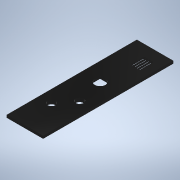
# Autodesk Inventor part: Arcade_ControlTop
Saved by Autodesk Inventor 2022 (Build 260153000, 153)
## iProperties
Created: 2023-12-22
Part Number: Arcade_ControlTop
Material: Generic
Document SubType Name: Modeling
Designer: Petr Černý
Density: 1 g/cm^3
Appearance: Smooth - Black
Author: Petr Černý
Autodesk Inventor part; units mm, degrees
ref_plane "YZ Plane" through (0, 0, 0) normal (1, 0, 0) x (0, 1, 0)
ref_plane "XZ Plane" through (0, 0, 0) normal (0, 1, 0) x (-1, 0, 0)
ref_plane "XY Plane" through (0, 0, 0) normal (0, 0, 1) x (1, 0, 0)
sketch "Sketch1" plane through (0, 0, 0) normal (0, 1, 0) x (-1, 0, 0)
  line L0 (23.5265, 54.5795) -> (-113.4735, 54.5795)
  line L1 (-113.4735, 54.5795) -> (-113.4735, -435.4205)
  line L2 (-113.4735, -435.4205) -> (23.5265, -435.4205)
  line L3 (23.5265, -435.4205) -> (23.5265, 54.5795)
  point P0 (0, 0)
  dimension "d0" = 137
  dimension "d1" = 490
  constraints: 8 end point, 2 parallel, 1 horizontal, 1 perpendicular
  measures "d0" distance of L2.end L1.end
  measures "d1" distance of L1.end L0.end
extrude "Extrusion1" add sketch "Sketch1" along normal blind 15
sketch "Sketch2" plane through (-23.5265, 0, 54.5795) normal (0, 0, 1) x (1, 0, 0)
  line L0 (137, 0) -> (0, 0) projected
  line L1 (0, 0) -> (127, 0)
  line L2 (127, 0) -> (127, 5)
  line L3 (127, 5) -> (0, 5)
  line L4 (0, 5) -> (0, 0)
  point P0 (23.5265, 0)
  dimension "d4" = 127
  dimension "d5" = 5
  constraints: 8 end point, 2 parallel, 1 horizontal, 1 perpendicular
  measures "d4" distance of L3.end L2.end
  measures "d5" distance of L2.end L1.end
extrude "Extrusion2" cut sketch "Sketch2" against normal blind 7
sketch "Sketch3" plane through (113.4735, 0, -435.4205) normal (0, 0, -1) x (-1, 0, 0)
  line L0 (0, 0) -> (137, 0) projected
  line L1 (0, 0) -> (137, 0)
  line L2 (137, 0) -> (137, 5)
  line L3 (137, 5) -> (0, 5)
  line L4 (0, 5) -> (0, 0)
  point P0 (113.4735, 0)
  dimension "d8" = 137
  dimension "d9" = 5
  constraints: 8 end point, 2 parallel, 1 horizontal, 1 perpendicular
  measures "d8" distance of L3.end L2.end
  measures "d9" distance of L2.end L1.end
extrude "Extrusion3" cut sketch "Sketch3" against normal blind 7
sketch "Sketch4" plane through (0, 0, 0) normal (0, -1, 0) x (1, 0, 0)
  line L0 (-23.5265, -428.4205) -> (113.4735, -428.4205) projected
  line L1 (103.4735, 47.5795) -> (-23.5265, 47.5795) projected
  line L2 (113.4735, -428.4205) -> (103.4735, -428.4205)
  line L3 (103.4735, -428.4205) -> (103.4735, 47.5795)
  line L4 (103.4735, 47.5795) -> (113.4735, 47.5795)
  line L5 (113.4735, 47.5795) -> (113.4735, -428.4205)
  point P0 (0, 0)
  point P1 (-13.5265, -428.4205)
  dimension "d12" = 10
  dimension "d13" = 476
  constraints: 8 end point, 2 parallel, 1 horizontal, 1 perpendicular
  measures "d12" distance of L1.start L4.end
  measures "d13" distance of L2.end L1.start
extrude "Extrusion4" cut sketch "Sketch4" against normal blind 5
sketch "Sketch5" plane through (0, 15, 0) normal (0, 1, 0) x (1, 0, 0)
  circle A0 centre (22.1402, 68.4205) radius 15
  circle A1 centre (67.8068, 128.4205) radius 15
  circle A2 centre (44.9735, 228.4205) radius 20
  line L0 (103.4735, 428.4205) -> (-23.5265, 428.4205) projected
  line L1 (-23.5265, 435.4205) -> (-23.5265, -54.5795) projected
  point P0 (0, 0)
  point P1 (-13.5265, 428.4205)
  dimension "d16" = 40
  dimension "d17" = 200
  dimension "d18" = 68.5
  dimension "d19" = 300
  dimension "d20" = 91.3333
  dimension "d21" = 45.6667
  dimension "d22" = 360
  dimension "d23" = 30
  dimension "d24" = 30
  constraints: 3 centre point
  measures "d16" diameter of A2
  measures "d17" distance from line of L0 A2.centre
  measures "d18" distance from line of A2.centre L1
  measures "d19" distance from line of L0 A1.centre
  measures "d20" distance from line of A1.centre L1
  measures "d21" distance from line of L1 A0.centre
  measures "d22" distance from line of L0 A0.centre
  measures "d23" diameter of A0
  measures "d24" diameter of A1
extrude "Extrusion5" cut sketch "Sketch5" against normal blind 15
sketch "Sketch6" plane through (0, 0, 0) normal (0, -1, 0) x (1, 0, 0)
  line L0 (69.9735, -253.4205) -> (19.9735, -253.4205)
  line L1 (19.9735, -253.4205) -> (19.9735, -203.4205)
  line L2 (19.9735, -203.4205) -> (69.9735, -203.4205)
  line L3 (69.9735, -203.4205) -> (69.9735, -253.4205)
  circle A0 centre (44.9735, -228.4205) radius 20 projected
  point P0 (0, 0)
  dimension "d27" = 25
  dimension "d28" = 50
  dimension "d29" = 25
  dimension "d30" = 50
  constraints: 8 end point, 2 parallel, 1 horizontal, 1 perpendicular
  measures "d27" distance from line of A0.centre L3
  measures "d28" distance of L0.start L0.end
  measures "d29" distance from line of L0 A0.centre
  measures "d30" distance between parallel lines of L2 L0
extrude "Extrusion6" cut sketch "Sketch6" against normal blind 12
sketch "Sketch7" plane through (0, 15, 0) normal (0, 1, 0) x (1, 0, 0)
  circle A0 centre (44.9735, 228.4205) radius 20 projected
  point P0 (0, 0)
  point P1 (28.7235, 212.1705)
  point P2 (28.7235, 244.6705)
  point P3 (61.2235, 244.6705)
  point P4 (61.2235, 212.1705)
  dimension "d33" = 16.25
  dimension "d34" = 16.25
  dimension "d35" = 16.25
  dimension "d36" = 16.25
  dimension "d37" = 16.25
  dimension "d38" = 16.25
  dimension "d39" = 16.25
  dimension "d40" = 16.25
  measures "d33" horizontal distance of A0.centre point (28.723, 212.17)
  measures "d34" horizontal distance of point (28.723, 244.67) A0.centre
  measures "d35" horizontal distance of A0.centre point (28.723, 244.67)
  measures "d36" horizontal distance of point (61.223, 244.67) A0.centre
  measures "d37" horizontal distance of A0.centre point (61.223, 244.67)
  measures "d38" horizontal distance of point (61.223, 212.17) A0.centre
  measures "d39" horizontal distance of A0.centre point (61.223, 212.17)
  measures "d40" horizontal distance of point (28.723, 212.17) A0.centre
hole "Hole1" at (28.7235, 15, -212.1705) at (28.7235, 15, -244.6705) at (61.2235, 15, -244.6705) at (61.2235, 15, -212.1705) direction (0, -1, 0) diameter 2.5 end through all
sketch "Sketch8" plane through (0, 0, 0) normal (0, -1, 0) x (1, 0, 0)
  circle A0 centre (61.2235, -244.6705) radius 1.25 projected
  circle A1 centre (28.7235, -212.1705) radius 1.25 projected
  circle A2 centre (28.7235, -244.6705) radius 1.25 projected
  circle A3 centre (61.2235, -212.1705) radius 1.25 projected
  line L0 (19.9735, -203.4205) -> (69.9735, -203.4205) projected
  line L1 (19.9735, -253.4205) -> (19.9735, -203.4205) projected
  line L2 (69.9735, -253.4205) -> (19.9735, -253.4205) projected
  line L3 (69.9735, -203.4205) -> (69.9735, -253.4205) projected
  circle A4 centre (44.9735, -228.4205) radius 20 projected
  line L4 (69.9735, -203.4205) -> (69.9735, -253.4205) projected
  line L5 (69.9735, -253.4205) -> (79.9735, -253.4205)
  line L6 (79.9735, -253.4205) -> (79.9735, -203.4205)
  line L7 (79.9735, -203.4205) -> (69.9735, -203.4205)
  line L8 (69.9735, -203.4205) -> (69.9735, -253.4205)
  line L9 (79.9735, -203.4205) -> (19.9735, -203.4205)
  line L10 (19.9735, -203.4205) -> (19.9735, -193.4205)
  line L11 (19.9735, -193.4205) -> (79.9735, -193.4205)
  line L12 (79.9735, -193.4205) -> (79.9735, -203.4205)
  point P0 (0, 0)
  dimension "d48" = 10
  dimension "d49" = 50
  dimension "d50" = 60
  dimension "d51" = 10
  constraints: 16 end point, 4 parallel, 2 horizontal, 2 perpendicular
  measures "d48" distance of L7.end L6.end
  measures "d49" distance of L6.end L5.end
  measures "d50" distance of L10.end L11.end
  measures "d51" distance of L9.end L10.end
extrude "Extrusion7" cut sketch "Sketch8" against normal blind 12 contours L10 L11 L12 L7 L0 | L7 L6 L5 L3
sketch "Sketch9" plane through (0, 15, 0) normal (0, 1, 0) x (1, 0, 0)
  line L0 (43.4735, 338.4205) -> (83.4735, 338.4205)
  line L1 (83.4735, 338.4205) -> (83.4735, 398.4205)
  line L2 (83.4735, 398.4205) -> (43.4735, 398.4205)
  line L3 (43.4735, 398.4205) -> (43.4735, 338.4205)
  line L4 (103.4735, 428.4205) -> (-23.5265, 428.4205) projected
  line L5 (113.4735, -54.5795) -> (113.4735, 435.4205) projected
  line L6 (46.6735, 342.9072) -> (52.6735, 342.9072)
  line L7 (52.6735, 342.9072) -> (52.6735, 392.9072)
  line L8 (52.6735, 392.9072) -> (46.6735, 392.9072)
  line L9 (46.6735, 392.9072) -> (46.6735, 342.9072)
  line L10 (55.8735, 342.9072) -> (61.8735, 342.9072)
  line L11 (61.8735, 342.9072) -> (61.8735, 392.9072)
  line L12 (61.8735, 392.9072) -> (55.8735, 392.9072)
  line L13 (55.8735, 392.9072) -> (55.8735, 342.9072)
  line L14 (65.0735, 342.9072) -> (71.0735, 342.9072)
  line L15 (71.0735, 342.9072) -> (71.0735, 392.9072)
  line L16 (71.0735, 392.9072) -> (65.0735, 392.9072)
  line L17 (65.0735, 392.9072) -> (65.0735, 342.9072)
  line L18 (74.2735, 342.9072) -> (80.2735, 342.9072)
  line L19 (80.2735, 342.9072) -> (80.2735, 392.9072)
  line L20 (80.2735, 392.9072) -> (74.2735, 392.9072)
  line L21 (74.2735, 392.9072) -> (74.2735, 342.9072)
  point P0 (0, 0)
  point P1 (-13.5265, 428.4205)
  dimension "d54" = 60
  dimension "d55" = 40
  dimension "d56" = 30
  dimension "d57" = 30
  dimension "d58" = 50
  dimension "d59" = 50
  dimension "d60" = 6
  dimension "d61" = 6
  dimension "d62" = 6
  dimension "d63" = 6
  dimension "d64" = 3.2
  dimension "d65" = 3.2
  dimension "d66" = 3.2
  dimension "d67" = 3.2
  constraints: 40 end point, 10 parallel, 5 horizontal, 5 perpendicular, 5 point on line
  measures "d54" distance of L2.end L0.start
  measures "d55" distance of L1.end L2.end
  measures "d56" distance between parallel lines of L4 L2
  measures "d57" distance between parallel lines of L5 L1
  measures "d58" distance of L8.end L6.start
  measures "d59" distance of L12.end L10.start
  measures "d60" distance of L7.end L8.end
  measures "d61" distance of L11.end L12.end
  measures "d62" distance of L15.end L16.end
  measures "d63" distance between parallel lines of L19 L21
  measures "d64" distance between parallel lines of L9 L3
  measures "d65" distance between parallel lines of L13 L7
  measures "d66" distance between parallel lines of L17 L11
  measures "d67" distance between parallel lines of L21 L15
extrude "Extrusion8" cut sketch "Sketch9" against normal blind 15 contours L9 L8 L7 L6 | L13 L12 L11 L10 | L17 L16 L15 L14 | L21 L20 L19 L18
sketch "Sketch11" plane through (0, 0, 0) normal (0, -1, 0) x (1, 0, 0)
  line L0 (103.4735, -400.4205) -> (23.4735, -400.4205)
  line L1 (23.4735, -400.4205) -> (23.4735, -285.4205)
  line L2 (23.4735, -285.4205) -> (103.4735, -285.4205)
  line L3 (103.4735, -285.4205) -> (103.4735, -400.4205)
  line L4 (113.4735, 47.5795) -> (113.4735, -435.4205) projected
  line L5 (113.4735, -435.4205) -> (-23.5265, -435.4205) projected
  point P0 (0, 0)
  point P1 (-13.5265, -435.4205)
  dimension "d70" = 80
  dimension "d71" = 115
  dimension "d72" = 10
  dimension "d73" = 35
  constraints: 8 end point, 2 parallel, 1 horizontal, 1 perpendicular
  measures "d70" distance of L1.end L2.end
  measures "d71" distance of L0.end L1.end
  measures "d72" distance between parallel lines of L4 L3
  measures "d73" distance between parallel lines of L5 L0
extrude "Extrusion9" cut sketch "Sketch11" against normal blind 10
sketch "Sketch12" plane through (-23.5265, 15, 54.5795) normal (0, 0, 1) x (1, 0, 0)
  line L0 (0, 0) -> (137, 0) projected
  line L1 (137, -121) -> (137, 0) projected
  line L2 (127, -15) -> (137, -15) projected
  line L3 (127, -10) -> (127, -121) projected
  line L4 (0, -10) -> (127, -10) projected
  line L5 (127, -10) -> (127, -121) projected
  line L6 (0, -10) -> (127, -10) projected
  line L7 (137, -15) -> (137, -10) projected
  line L8 (127, -10) -> (137, -10)
  line L9 (137, -10) -> (137, -15)
  line L10 (137, -15) -> (127, -15)
  line L11 (127, -15) -> (127, -10)
  point P0 (23.5265, -15)
  constraints: 8 end point, 2 parallel, 1 perpendicular
extrude "Extrusion10" cut sketch "Sketch12" against normal blind 7
body "Solid1"
